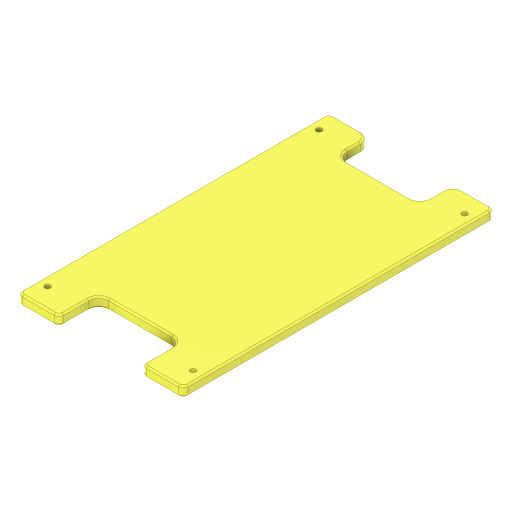
# Autodesk Inventor part: Cathode-Cover-Plate-bottom-side
Saved by Autodesk Inventor 2024.2 (Build 282272000, 272)
## iProperties
Created: 2023-12-01
Part Number: Cathode-Cover-Plate-bottom-side
Material: Generic
Document SubType Name: Modeling
Designer: kuzmin
Density: 1 g/cm^3
Appearance: Smooth - Yellow
Author: kuzmin
Autodesk Inventor part; units mm, degrees
ref_plane "YZ Plane" through (0, 0, 0) normal (1, 0, 0) x (0, 1, 0)
ref_plane "XZ Plane" through (0, 0, 0) normal (0, 1, 0) x (-1, 0, 0)
ref_plane "XY Plane" through (0, 0, 0) normal (0, 0, 1) x (1, 0, 0)
sketch "Sketch1" plane through (0, 0, 0) normal (0, 0, 1) x (1, 0, 0)
  line L0 (-94, 50) -> (94, 50)
  line L1 (94, 50) -> (94, -50)
  line L2 (94, -50) -> (-94, -50)
  line L3 (-94, -50) -> (-94, 50)
  point P0 (0, 0)
  point P1 (0, 50)
  point P2 (94, 0)
  dimension "d2" = 100
  dimension "d3" = 188
  constraints: 8 end point, 2 midpoint, 2 parallel, 1 horizontal, 1 horizontal alignment, 1 perpendicular, 1 vertical alignment
  measures "d2" distance of L0.end L1.end
  measures "d3" distance of L0.start L0.end
extrude "Extrusion1" add sketch "Sketch1" along normal blind 6
sketch "Sketch5" plane through (0, 0, 6) normal (0, 0, 1) x (1, 0, 0)
  circle A0 centre (82, -43.9615) radius 1.7
  circle A1 centre (82, 43.9615) radius 1.7
  line L0 (82, -43.9615) -> (82, 43.9615) construction
  line L1 (94, -50) -> (94, 50) projected
  point P0 (0, 0)
  point P1 (82, 0)
  point P2 (94, 0)
  dimension "d27" = 3.4
  dimension "d28" = 12
  dimension "d29" = 87.923
  constraints: 2 centre point, 2 end point, 2 midpoint, 1 equal radius, 1 horizontal alignment, 1 vertical
  measures "d27" diameter of A0
  measures "d28" distance between parallel lines of L1 L0
  measures "d29" distance of L0.start L0.end
extrude "Extrusion5" cut sketch "Sketch5" against normal through all
sketch "Sketch6" plane through (0, 0, 6) normal (0, 0, 1) x (1, 0, 0)
  line L0 (70, 25) -> (94, 25)
  line L1 (94, 25) -> (94, -25)
  line L2 (94, -25) -> (70, -25)
  line L3 (70, -25) -> (70, 25)
  line L4 (94, -50) -> (94, 50) projected
  point P0 (0, 0)
  point P1 (94, 0)
  dimension "d34" = 24
  dimension "d35" = 50
  constraints: 8 end point, 2 midpoint, 2 parallel, 1 horizontal, 1 perpendicular
  measures "d34" distance of L0.start L0.end
  measures "d35" distance of L2.end L0.start
extrude "Extrusion6" cut sketch "Sketch6" against normal through all
fillet "Fillet2" radius 6 2 edges at (70, -25, 3) (70, 25, 3)
fillet "Fillet3" radius 3 6 edges at (94, -25, 3) (94, -50, 3) (94, 25, 3) (94, 50, 3) (-94, 50, 3) (-94, -50, 3)
sketch "Sketch9" plane through (0, 0, 6) normal (0, 0, 1) x (1, 0, 0)
  circle A0 centre (-82, 43.9615) radius 1.7
  circle A1 centre (-82, -43.9615) radius 1.7
  line L0 (-82, -43.9615) -> (-82, 43.9615) construction
  line L1 (-94, 47) -> (-94, -47) projected
  point P0 (0, 0)
  point P1 (-82, 0)
  point P2 (-94, 0)
  dimension "d47" = 87.923
  dimension "d48" = 12
  dimension "d49" = 3.4
  constraints: 2 centre point, 2 end point, 2 midpoint, 1 equal radius, 1 horizontal alignment, 1 vertical
  measures "d47" distance of L0.start L0.end
  measures "d48" distance between parallel lines of L1 L0
  measures "d49" diameter of A0
extrude "Extrusion8" cut sketch "Sketch9" against normal through all
sketch "Sketch10" plane through (0, 0, 6) normal (0, 0, 1) x (1, 0, 0)
  line L0 (-94, 47) -> (-94, -47) projected
  line L1 (-94, -25) -> (-74, -25)
  line L2 (-74, -25) -> (-74, 25)
  line L3 (-74, 25) -> (-94, 25)
  line L4 (-94, 25) -> (-94, -25)
  point P0 (0, 0)
  point P1 (-94, 0)
  dimension "d52" = 50
  dimension "d53" = 20
  constraints: 8 end point, 2 midpoint, 2 parallel, 1 horizontal, 1 perpendicular, 1 point on line
  measures "d52" distance of L1.end L2.end
  measures "d53" distance of L2.end L3.end
extrude "Extrusion9" cut sketch "Sketch10" against normal through all
fillet "Fillet4" radius 6 4 edges at (-74, -25, 3) (-74, 25, 3) (-94, -25, 3) (-94, 25, 3)
chamfer "Chamfer5" distance 1 angle 45 48 edges at (0, -50, 6) (93.1213, -49.1213, 6) (94, -37.5, 6) (93.1213, -25.8787, 6) (83.5, -25, 6) (71.7574, -23.2426, 6) (70, 0, 6) (71.7574, 23.2426, 6) (83.5, 25, 6) (93.1213, 25.8787, 6) (94, 37.5, 6) (93.1213, 49.1213, 6) (0, 50, 6) (-93.1213, 49.1213, 6) (-94, 39, 6) (-92.2426, 26.7574, 6) (-84, 25, 6) (-75.7574, 23.2426, 6) (-74, 0, 6) (-75.7574, -23.2426, 6) (-84, -25, 6) (-92.2426, -26.7574, 6) (-94, -39, 6) (-93.1213, -49.1213, 6) (0, 50, 0) (-93.1213, 49.1213, 0) (-94, 39, 0) (-92.2426, 26.7574, 0) (-84, 25, 0) (-75.7574, 23.2426, 0) (-74, 0, 0) (-75.7574, -23.2426, 0) (-84, -25, 0) (-92.2426, -26.7574, 0) (-94, -39, 0) (-93.1213, -49.1213, 0) (0, -50, 0) (93.1213, -49.1213, 0) (94, -37.5, 0) (93.1213, -25.8787, 0) (83.5, -25, 0) (71.7574, -23.2426, 0) (70, 0, 0) (71.7574, 23.2426, 0) (83.5, 25, 0) (93.1213, 25.8787, 0) (94, 37.5, 0) (93.1213, 49.1213, 0)
body "Solid1"
